Autodesk Fusion 360 part; units mm, degrees
(part 3 of 4)
sketch "v3" plane through (0, 0, 0) normal (0, 1, 0) x (1, 0, 0)
  line L0 (97.775, -35.41) -> (97.775, -48.41)
  arc A0 (111.775, -54.46) -> (111.275, -53.96) centre (111.275, -54.46) ccw
  arc A1 (68.5566, -88.749) -> (70.5283, -89.9625) centre (70.9931, -86.9987) ccw
  arc A2 (98.275, -34.91) -> (97.775, -35.41) centre (98.275, -35.41) ccw
  arc A3 (92.725, -52.555) -> (92.225, -52.055) centre (92.225, -52.555) ccw
  arc A4 (79.225, -52.055) -> (78.725, -52.555) centre (79.225, -52.555) ccw
  arc A5 (92.225, -47.005) -> (92.725, -46.505) centre (92.225, -46.505) ccw
  arc A6 (73.175, -56.53) -> (73.675, -56.03) centre (73.175, -56.03) ccw
  line L1 (92.225, -52.555) -> (92.225, -46.505) construction
  line L2 (79.225, -47.005) -> (92.225, -47.005)
  arc A7 (2.525, -73.175) -> (3.025, -73.675) centre (3.025, -73.175) ccw
  line L3 (113.775, -14.86) -> (113.775, -16.36)
  arc A8 (54.125, -24.145) -> (54.625, -23.645) centre (54.125, -23.645) ccw
  line L4 (22.075, -33.67) -> (35.075, -33.67)
  arc A9 (111.775, -16.36) -> (111.275, -15.86) centre (111.275, -16.36) ccw
  arc A10 (73.175, -18.43) -> (73.675, -17.93) centre (73.175, -17.93) ccw
  arc A11 (40.625, -42.695) -> (41.125, -43.195) centre (41.125, -42.695) ccw
  line L5 (35.575, -20.17) -> (35.575, -33.17)
  arc A12 (21.575, -33.17) -> (22.075, -33.67) centre (22.075, -33.17) ccw
  arc A13 (120.896, -78.4821) -> (120.213, -78.6651) centre (120.646, -78.9151) ccw
  line L6 (40.625, -10.645) -> (40.625, -23.645)
  line L7 (59.675, -23.98) -> (59.675, -36.98)
  line L8 (79.225, -66.055) -> (92.225, -66.055)
  arc A14 (113.775, -14.86) -> (112.775, -13.86) centre (112.775, -14.86) ccw
  arc A15 (40.625, -61.745) -> (41.125, -62.245) centre (41.125, -61.745) ccw
  line L9 (68.5566, -88.749) -> (60.0623, -76.9247)
  line L10 (22.075, -35.075) -> (22.075, -41.125) construction
  line L11 (22.075, -41.125) -> (16.025, -41.125) construction
  arc A16 (109.3213, -79.6939) -> (108.9677, -79.0815) centre (108.8383, -79.5645) ccw
  line L12 (22.075, -57.77) -> (35.075, -57.77)
  arc A17 (113.775, -65.0177) -> (115.275, -67.6158) centre (116.775, -65.0177) ccw
  arc A18 (41.125, -29.195) -> (40.625, -29.695) centre (41.125, -29.695) ccw
  line L13 (41.125, -43.195) -> (54.125, -43.195)
  arc A19 (94.725, -13.36) -> (95.225, -13.86) centre (95.225, -13.36) ccw
  arc A20 (35.575, -39.22) -> (35.075, -38.72) centre (35.075, -39.22) ccw
  arc A21 (40.625, -23.645) -> (41.125, -24.145) centre (41.125, -23.645) ccw
  arc A22 (92.4336, -88.6274) -> (92.7872, -89.2398) centre (92.9166, -88.7568) ccw
  line L14 (136.7533, -80.0163) -> (115.275, -67.6158)
  arc A23 (54.125, -62.245) -> (54.625, -61.745) centre (54.125, -61.745) ccw
  line L15 (21.575, -20.17) -> (21.575, -33.17)
  line L16 (22.075, -19.67) -> (35.075, -19.67)
  arc A24 (60.175, -23.48) -> (59.675, -23.98) centre (60.175, -23.98) ccw
  line L17 (94.725, -12.455) -> (94.725, -13.36)
  arc A25 (92.225, -66.055) -> (92.725, -65.555) centre (92.225, -65.555) ccw
  line L18 (73.675, -4.93) -> (73.675, -17.93)
  arc A26 (60.175, -4.43) -> (59.675, -4.93) centre (60.175, -4.93) ccw
  arc A27 (85.5575, -87.9625) -> (86.0575, -87.4625) centre (85.5575, -87.4625) ccw
  arc A28 (3.025, -40.625) -> (2.525, -41.125) centre (3.025, -41.125) ccw
  line L19 (35.575, -58.27) -> (35.575, -71.27)
  line L20 (75.175, -2.43) -> (73.175, -2.43)
  arc A29 (3.025, -21.575) -> (2.525, -22.075) centre (3.025, -22.075) ccw
  line L21 (107.725, -13.86) -> (112.775, -13.86)
  line L22 (57.675, -7.645) -> (57.675, -2.93)
  arc A30 (54.625, -48.745) -> (54.125, -48.245) centre (54.125, -48.745) ccw
  arc A31 (94.725, -12.455) -> (94.225, -11.955) centre (94.225, -12.455) ccw
  arc A32 (57.175, -8.145) -> (57.675, -7.645) centre (57.175, -7.645) ccw
  arc A33 (2.525, -54.125) -> (3.025, -54.625) centre (3.025, -54.125) ccw
  arc A34 (60.175, -42.53) -> (59.675, -43.03) centre (60.175, -43.03) ccw
  line L23 (41.125, -24.145) -> (54.125, -24.145)
  circle A35 centre (66.675, -65.625) radius 1
  line L24 (120.213, -78.6651) -> (113.713, -89.9234)
  line L25 (3.025, -54.625) -> (16.025, -54.625)
  arc A36 (54.625, -10.645) -> (54.125, -10.145) centre (54.125, -10.645) ccw
  line L26 (125.1543, -97.1064) -> (113.896, -90.6064)
  line L27 (72.5575, -73.9625) -> (85.5575, -73.9625)
  line L28 (3.025, -35.575) -> (16.025, -35.575)
  arc A37 (73.675, -4.93) -> (73.175, -4.43) centre (73.175, -4.93) ccw
  arc A38 (54.625, -29.695) -> (54.125, -29.195) centre (54.125, -29.695) ccw
  line L29 (86.0575, -74.4625) -> (86.0575, -87.4625)
  arc A39 (35.075, -33.67) -> (35.575, -33.17) centre (35.075, -33.17) ccw
  line L30 (22.075, -38.72) -> (35.075, -38.72)
  arc A40 (132.3373, -85.6651) -> (132.1543, -84.9821) centre (131.9043, -85.4151) ccw
  line L31 (0.525, -22.075) -> (0.525, -35.075)
  line L32 (41.125, -29.195) -> (54.125, -29.195)
  arc A41 (79.225, -13.955) -> (78.725, -14.455) centre (79.225, -14.455) ccw
  line L33 (54.625, -29.695) -> (54.625, -42.695)
  line L34 (70.5283, -89.9625) -> (109.8625, -96.1307)
  line L35 (59.675, -43.03) -> (59.675, -56.03)
  line L36 (25.625, -17.67) -> (38.125, -17.67)
  line L37 (92.7872, -89.2398) -> (105.3442, -92.6045)
  line L38 (98.275, -67.96) -> (111.275, -67.96)
  circle A42 centre (95.25, -49.53) radius 1
  line L39 (113.775, -16.36) -> (113.775, -29.36)
  line L40 (97.775, -54.46) -> (97.775, -67.46)
  line L41 (95.7983, -76.0704) -> (92.4336, -88.6274)
  line L42 (92.725, -14.455) -> (92.725, -27.455)
  line L43 (16.025, -35.075) -> (22.075, -35.075) construction
  line L44 (73.675, -23.98) -> (73.675, -36.98)
  line L45 (132.1543, -84.9821) -> (120.896, -78.4821)
  line L46 (22.075, -71.77) -> (35.075, -71.77)
  line L47 (0.525, -41.125) -> (0.525, -54.125)
  line L48 (16.525, -41.125) -> (16.525, -54.125)
  line L49 (98.275, -33.505) -> (92.225, -33.505) construction
  line L50 (2.525, -41.125) -> (2.525, -54.125)
  line L51 (97.775, -16.36) -> (97.775, -29.36)
  line L52 (40.625, -29.695) -> (40.625, -42.695)
  line L53 (111.775, -16.36) -> (111.775, -29.36)
  line L54 (98.275, -52.555) -> (92.225, -52.555) construction
  line L55 (22.075, -52.72) -> (35.075, -52.72)
  line L56 (78.725, -14.455) -> (78.725, -27.455)
  line L57 (92.225, -27.455) -> (98.275, -27.455) construction
  line L58 (96.4107, -75.7169) -> (108.9677, -79.0815)
  line L59 (132.1543, -84.9821) -> (120.896, -78.4821)
  line L60 (20.075, -17.67) -> (25.625, -17.67)
  arc A43 (137.1194, -81.3823) -> (136.7533, -80.0163) centre (136.2533, -80.8823) ccw
  line L61 (88.675, -11.955) -> (94.225, -11.955)
  line L62 (22.075, -71.77) -> (35.075, -71.77)
  arc A44 (111.275, -67.96) -> (111.775, -67.46) centre (111.275, -67.46) ccw
  arc A45 (97.775, -67.46) -> (98.275, -67.96) centre (98.275, -67.46) ccw
  line L63 (54.625, -10.645) -> (54.625, -23.645)
  line L64 (16.025, -75.675) -> (57.6258, -75.675)
  line L65 (39.125, -8.145) -> (44.675, -8.145)
  arc A46 (35.575, -58.27) -> (35.075, -57.77) centre (35.075, -58.27) ccw
  arc A47 (41.125, -10.145) -> (40.625, -10.645) centre (41.125, -10.645) ccw
  line L66 (19.575, -19.075) -> (19.575, -18.17)
  arc A48 (19.075, -19.575) -> (19.575, -19.075) centre (19.075, -19.075) ccw
  line L67 (41.125, -48.245) -> (54.125, -48.245)
  line L68 (58.175, -2.43) -> (60.175, -2.43)
  arc A49 (16.525, -22.075) -> (16.025, -21.575) centre (16.025, -22.075) ccw
  line L69 (40.625, -48.745) -> (40.625, -61.745)
  arc A50 (41.125, -48.245) -> (40.625, -48.745) centre (41.125, -48.745) ccw
  line L70 (137.1194, -81.3823) -> (127.5694, -97.9234)
  circle A51 centre (19.05, -38.1) radius 1
  line L71 (22.075, -54.125) -> (22.075, -60.175) construction
  arc A52 (125.1543, -97.1064) -> (125.8373, -96.9234) centre (125.4043, -96.6734) ccw
  arc A53 (123.1533, -103.5722) -> (124.5194, -103.2062) centre (123.6533, -102.7062) ccw
  line L72 (132.3373, -85.6651) -> (125.8373, -96.9234)
  arc A54 (16.525, -41.125) -> (16.025, -40.625) centre (16.025, -41.125) ccw
  line L73 (0.525, -60.175) -> (0.525, -74.675)
  arc A55 (21.575, -52.22) -> (22.075, -52.72) centre (22.075, -52.22) ccw
  line L74 (2.525, -60.175) -> (2.525, -73.175)
  arc A56 (16.525, -60.175) -> (16.025, -59.675) centre (16.025, -60.175) ccw
  arc A57 (75.675, -11.455) -> (76.175, -11.955) centre (76.175, -11.455) ccw
  line L75 (16.025, -41.125) -> (16.025, -35.075) construction
  line L76 (0.525, -22.075) -> (0.525, -20.575)
  line L77 (2.525, -22.075) -> (2.525, -35.075)
  line L78 (54.625, -48.745) -> (54.625, -61.745)
  line L79 (6.575, -19.575) -> (19.075, -19.575)
  line L80 (16.525, -60.175) -> (16.525, -73.175)
  arc A58 (35.075, -71.77) -> (35.575, -71.27) centre (35.075, -71.27) ccw
  line L81 (22.075, -60.175) -> (16.025, -60.175) construction
  line L82 (3.025, -73.675) -> (16.025, -73.675)
  line L83 (0.525, -60.175) -> (0.525, -54.125)
  line L84 (16.025, -60.175) -> (16.025, -54.125) construction
  line L85 (3.025, -21.575) -> (16.025, -21.575)
  arc A59 (16.025, -73.675) -> (16.525, -73.175) centre (16.025, -73.175) ccw
  line L86 (1.525, -19.575) -> (3.025, -19.575)
  arc A60 (21.575, -71.27) -> (22.075, -71.77) centre (22.075, -71.27) ccw
  line L87 (6.575, -19.575) -> (3.025, -19.575)
  line L88 (2.525, -60.175) -> (2.525, -73.175)
  arc A61 (3.025, -59.675) -> (2.525, -60.175) centre (3.025, -60.175) ccw
  arc A62 (0.525, -74.675) -> (1.525, -75.675) centre (1.525, -74.675) ccw
  line L89 (1.525, -75.675) -> (16.025, -75.675)
  arc A63 (1.525, -19.575) -> (0.525, -20.575) centre (1.525, -20.575) ccw
  arc A64 (20.075, -17.67) -> (19.575, -18.17) centre (20.075, -18.17) ccw
  arc A65 (78.725, -65.555) -> (79.225, -66.055) centre (79.225, -65.555) ccw
  arc A66 (16.025, -35.575) -> (16.525, -35.075) centre (16.025, -35.075) ccw
  line L90 (75.675, -11.455) -> (75.675, -2.93)
  arc A67 (39.125, -8.145) -> (38.625, -8.645) centre (39.125, -8.645) ccw
  line L91 (0.525, -41.125) -> (0.525, -35.075)
  line L92 (59.675, -4.93) -> (59.675, -17.93)
  arc A68 (113.713, -89.9234) -> (113.896, -90.6064) centre (114.146, -90.1734) ccw
  arc A69 (72.0575, -87.4625) -> (72.5575, -87.9625) centre (72.5575, -87.4625) ccw
  arc A70 (22.075, -38.72) -> (21.575, -39.22) centre (22.075, -39.22) ccw
  arc A71 (59.675, -36.98) -> (60.175, -37.48) centre (60.175, -36.98) ccw
  arc A72 (22.075, -19.67) -> (21.575, -20.17) centre (22.075, -20.17) ccw
  arc A73 (59.675, -17.93) -> (60.175, -18.43) centre (60.175, -17.93) ccw
  arc A74 (16.025, -54.625) -> (16.525, -54.125) centre (16.025, -54.125) ccw
  arc A75 (38.125, -17.67) -> (38.625, -17.17) centre (38.125, -17.17) ccw
  arc A76 (35.075, -52.72) -> (35.575, -52.22) centre (35.075, -52.22) ccw
  line L93 (38.625, -17.17) -> (38.625, -8.645)
  arc A77 (86.0575, -74.4625) -> (85.5575, -73.9625) centre (85.5575, -74.4625) ccw
  line L94 (41.125, -62.245) -> (54.125, -62.245)
  line L95 (72.0575, -74.4625) -> (72.0575, -87.4625)
  arc A78 (60.0623, -76.9247) -> (57.6258, -75.675) centre (57.6258, -78.675) ccw
  circle A79 centre (19.05, -57.15) radius 1
  line L96 (76.175, -11.955) -> (88.675, -11.955)
  line L97 (41.125, -62.245) -> (54.125, -62.245)
  line L98 (123.1533, -103.5722) -> (110.8977, -96.4964)
  line L99 (44.675, -8.145) -> (57.175, -8.145)
  line L100 (72.0575, -74.4625) -> (72.0575, -87.4625)
  arc A80 (22.075, -57.77) -> (21.575, -58.27) centre (22.075, -58.27) ccw
  line L101 (3.025, -40.625) -> (16.025, -40.625)
  arc A81 (105.3442, -92.6045) -> (105.9566, -92.2509) centre (105.4736, -92.1215) ccw
  arc A82 (35.575, -20.17) -> (35.075, -19.67) centre (35.075, -20.17) ccw
  arc A83 (98.275, -15.86) -> (97.775, -16.36) centre (98.275, -16.36) ccw
  line L102 (79.225, -13.955) -> (92.225, -13.955)
  line L103 (109.3213, -79.6939) -> (105.9566, -92.2509)
  line L104 (98.275, -15.86) -> (111.275, -15.86)
  arc A84 (59.675, -56.03) -> (60.175, -56.53) centre (60.175, -56.03) ccw
  arc A85 (96.4107, -75.7169) -> (95.7983, -76.0704) centre (96.2813, -76.1998) ccw
  line L105 (41.125, -10.145) -> (54.125, -10.145)
  line L106 (16.025, -54.125) -> (22.075, -54.125) construction
  line L107 (21.575, -58.27) -> (21.575, -71.27)
  arc A86 (110.8977, -96.4964) -> (109.8625, -96.1307) centre (109.3977, -99.0945) ccw
  line L108 (95.225, -13.86) -> (107.725, -13.86)
  line L109 (16.525, -22.075) -> (16.525, -35.075)
  arc A87 (54.125, -43.195) -> (54.625, -42.695) centre (54.125, -42.695) ccw
  arc A88 (72.5575, -73.9625) -> (72.0575, -74.4625) centre (72.5575, -74.4625) ccw
  line L110 (3.025, -59.675) -> (16.025, -59.675)
  arc A89 (2.525, -35.075) -> (3.025, -35.575) centre (3.025, -35.075) ccw
  line L111 (72.5575, -87.9625) -> (85.5575, -87.9625)
  line L112 (124.5194, -103.2062) -> (127.5694, -97.9234)
  arc A90 (92.725, -14.455) -> (92.225, -13.955) centre (92.225, -14.455) ccw
  arc A91 (75.675, -2.93) -> (75.175, -2.43) centre (75.175, -2.93) ccw
  line L113 (66.675, -47.625) -> (66.675, -65.625) construction
  arc A92 (58.175, -2.43) -> (57.675, -2.93) centre (58.175, -2.93) ccw
  arc A93 (73.675, -23.98) -> (73.175, -23.48) centre (73.175, -23.98) ccw
  arc A94 (111.275, -48.91) -> (111.775, -48.41) centre (111.275, -48.41) ccw
  arc A95 (97.775, -29.36) -> (98.275, -29.86) centre (98.275, -29.36) ccw
  line L114 (98.275, -27.455) -> (98.275, -33.505) construction
  line L115 (111.775, -35.41) -> (111.775, -48.41)
  arc A96 (111.275, -29.86) -> (111.775, -29.36) centre (111.275, -29.36) ccw
  line L116 (98.275, -29.86) -> (111.275, -29.86)
  line L117 (98.275, -46.505) -> (98.275, -52.555) construction
  line L118 (98.275, -53.96) -> (111.275, -53.96)
  line L119 (98.275, -48.91) -> (111.275, -48.91)
  line L120 (98.275, -34.91) -> (111.275, -34.91)
  line L121 (113.775, -54.46) -> (113.775, -48.41)
  arc A97 (98.275, -53.96) -> (97.775, -54.46) centre (98.275, -54.46) ccw
  line L122 (113.775, -35.41) -> (113.775, -29.36)
  arc A98 (111.775, -35.41) -> (111.275, -34.91) centre (111.275, -35.41) ccw
  line L123 (113.775, -35.41) -> (113.775, -48.41)
  arc A99 (97.775, -48.41) -> (98.275, -48.91) centre (98.275, -48.41) ccw
  line L124 (79.225, -27.955) -> (92.225, -27.955)
  arc A100 (78.725, -27.455) -> (79.225, -27.955) centre (79.225, -27.455) ccw
  line L125 (79.225, -33.005) -> (92.225, -33.005)
  line L126 (60.175, -2.43) -> (73.175, -2.43)
  arc A101 (79.225, -33.005) -> (78.725, -33.505) centre (79.225, -33.505) ccw
  line L127 (113.775, -54.46) -> (113.775, -65.0177)
  line L128 (92.725, -52.555) -> (92.725, -65.555)
  line L129 (2.525, -41.125) -> (2.525, -54.125)
  line L130 (78.725, -52.555) -> (78.725, -65.555)
  line L131 (92.225, -33.505) -> (92.225, -27.455) construction
  line L132 (92.225, -46.505) -> (98.275, -46.505) construction
  circle A102 centre (95.25, -30.48) radius 1
  line L133 (111.775, -54.46) -> (111.775, -67.46)
  arc A103 (92.225, -27.955) -> (92.725, -27.455) centre (92.225, -27.455) ccw
  line L134 (73.675, -43.03) -> (73.675, -56.03)
  line L135 (35.575, -39.22) -> (35.575, -52.22)
  line L136 (21.575, -39.22) -> (21.575, -52.22)
  line L137 (60.175, -18.43) -> (73.175, -18.43)
  arc A104 (92.725, -33.505) -> (92.225, -33.005) centre (92.225, -33.505) ccw
  line L138 (60.175, -23.48) -> (73.175, -23.48)
  line L139 (79.225, -52.055) -> (92.225, -52.055)
  line L140 (78.725, -33.505) -> (78.725, -46.505)
  arc A105 (73.175, -37.48) -> (73.675, -36.98) centre (73.175, -36.98) ccw
  arc A106 (78.725, -46.505) -> (79.225, -47.005) centre (79.225, -46.505) ccw
  line L141 (60.175, -37.48) -> (73.175, -37.48)
  line L142 (60.175, -42.53) -> (73.175, -42.53)
  arc A107 (73.675, -43.03) -> (73.175, -42.53) centre (73.175, -43.03) ccw
  line L143 (60.175, -56.53) -> (73.175, -56.53)
  line L144 (60.175, -4.43) -> (73.175, -4.43)
  line L145 (92.725, -33.505) -> (92.725, -46.505)
  line L146 (150, 0) -> (150, -125) construction
  line L147 (179.787, -78.6651) -> (186.287, -89.9234)
  line L148 (167.8457, -84.9821) -> (179.104, -78.4821)
  line L149 (190.6787, -79.6939) -> (194.0434, -92.2509)
  line L150 (162.8806, -81.3823) -> (172.4306, -97.9234)
  line L151 (167.8457, -84.9821) -> (179.104, -78.4821)
  line L152 (239.825, -4.43) -> (226.825, -4.43)
  line L153 (239.825, -2.43) -> (226.825, -2.43)
  arc A108 (204.2017, -76.0704) -> (203.5893, -75.7169) centre (203.7187, -76.1998) ccw
  arc A109 (207.2128, -89.2398) -> (207.5664, -88.6274) centre (207.0834, -88.7568) ccw
  line L154 (239.825, -42.53) -> (226.825, -42.53)
  arc A110 (229.4717, -89.9625) -> (231.4434, -88.749) centre (229.0069, -86.9987) ccw
  arc A111 (207.275, -65.555) -> (207.775, -66.055) centre (207.775, -65.555) ccw
  arc A112 (213.9425, -87.4625) -> (214.4425, -87.9625) centre (214.4425, -87.4625) ccw
  circle A113 centre (204.75, -49.53) radius 1
  arc A114 (202.225, -16.36) -> (201.725, -15.86) centre (201.725, -16.36) ccw
  line L155 (201.725, -27.455) -> (201.725, -33.505) construction
  line L156 (205.275, -12.455) -> (205.275, -13.36)
  line L157 (226.325, -43.03) -> (226.325, -56.03)
  line L158 (224.325, -11.455) -> (224.325, -2.93)
  arc A115 (188.725, -15.86) -> (188.225, -16.36) centre (188.725, -16.36) ccw
  arc A116 (205.775, -11.955) -> (205.275, -12.455) centre (205.775, -12.455) ccw
  arc A117 (207.275, -27.455) -> (207.775, -27.955) centre (207.775, -27.455) ccw
  arc A118 (204.775, -13.86) -> (205.275, -13.36) centre (204.775, -13.36) ccw
  line L159 (207.775, -27.455) -> (201.725, -27.455) construction
  line L160 (220.775, -47.005) -> (207.775, -47.005)
  line L161 (188.225, -35.41) -> (188.225, -48.41)
  line L162 (192.275, -13.86) -> (187.225, -13.86)
  line L163 (298.475, -19.575) -> (296.975, -19.575)
  arc A119 (259.375, -48.745) -> (258.875, -48.245) centre (258.875, -48.745) ccw
  line L164 (201.725, -15.86) -> (188.725, -15.86)
  line L165 (283.475, -60.175) -> (283.475, -73.175)
  arc A120 (201.725, -48.91) -> (202.225, -48.41) centre (201.725, -48.41) ccw
  line L166 (298.475, -75.675) -> (283.975, -75.675)
  arc A121 (188.725, -53.96) -> (188.225, -54.46) centre (188.725, -54.46) ccw
  line L167 (186.225, -14.86) -> (186.225, -16.36)
  arc A122 (187.225, -13.86) -> (186.225, -14.86) centre (187.225, -14.86) ccw
  line L168 (299.475, -60.175) -> (299.475, -74.675)
  line L169 (201.725, -53.96) -> (188.725, -53.96)
  line L170 (224.825, -2.43) -> (226.825, -2.43)
  line L171 (226.325, -4.93) -> (226.325, -17.93)
  arc A123 (201.725, -29.86) -> (202.225, -29.36) centre (201.725, -29.36) ccw
  arc A124 (226.825, -23.48) -> (226.325, -23.98) centre (226.825, -23.98) ccw
  arc A125 (224.825, -2.43) -> (224.325, -2.93) centre (224.825, -2.93) ccw
  line L172 (223.825, -11.955) -> (211.325, -11.955)
  arc A126 (277.925, -52.72) -> (278.425, -52.22) centre (277.925, -52.22) ccw
  arc A127 (207.275, -46.505) -> (207.775, -47.005) centre (207.775, -46.505) ccw
  line L173 (201.725, -34.91) -> (188.725, -34.91)
  arc A128 (226.825, -4.43) -> (226.325, -4.93) centre (226.825, -4.93) ccw
  arc A129 (223.825, -11.955) -> (224.325, -11.455) centre (223.825, -11.455) ccw
  circle A130 centre (280.95, -57.15) radius 1
  line L174 (201.725, -46.505) -> (201.725, -52.555) construction
  line L175 (283.975, -54.125) -> (277.925, -54.125) construction
  line L176 (220.775, -52.055) -> (207.775, -52.055)
  line L177 (220.775, -13.955) -> (207.775, -13.955)
  arc A131 (207.775, -13.955) -> (207.275, -14.455) centre (207.775, -14.455) ccw
  line L178 (296.975, -59.675) -> (283.975, -59.675)
  line L179 (296.975, -54.625) -> (283.975, -54.625)
  arc A132 (221.275, -14.455) -> (220.775, -13.955) centre (220.775, -14.455) ccw
  arc A133 (226.325, -17.93) -> (226.825, -18.43) centre (226.825, -17.93) ccw
  line L180 (207.275, -33.505) -> (207.275, -46.505)
  arc A134 (296.975, -54.625) -> (297.475, -54.125) centre (296.975, -54.125) ccw
  arc A135 (226.825, -42.53) -> (226.325, -43.03) centre (226.825, -43.03) ccw
  arc A136 (283.475, -54.125) -> (283.975, -54.625) centre (283.975, -54.125) ccw
  arc A137 (220.775, -27.955) -> (221.275, -27.455) centre (220.775, -27.455) ccw
  arc A138 (278.425, -58.27) -> (277.925, -57.77) centre (277.925, -58.27) ccw
  arc A139 (283.475, -73.175) -> (283.975, -73.675) centre (283.975, -73.175) ccw
  arc A140 (239.825, -56.53) -> (240.325, -56.03) centre (239.825, -56.03) ccw
  arc A141 (280.425, -18.17) -> (279.925, -17.67) centre (279.925, -18.17) ccw
  line L181 (201.725, -33.505) -> (207.775, -33.505) construction
  line L182 (186.225, -35.41) -> (186.225, -29.36)
  line L183 (299.475, -22.075) -> (299.475, -35.075)
  arc A142 (299.475, -20.575) -> (298.475, -19.575) centre (298.475, -20.575) ccw
  circle A143 centre (280.95, -38.1) radius 1
  line L184 (277.925, -60.175) -> (283.975, -60.175) construction
  circle A144 centre (204.75, -30.48) radius 1
  line L185 (297.475, -22.075) -> (297.475, -35.075)
  line L186 (201.725, -52.555) -> (207.775, -52.555) construction
  arc A145 (283.475, -35.075) -> (283.975, -35.575) centre (283.975, -35.075) ccw
  line L187 (280.425, -19.075) -> (280.425, -18.17)
  arc A146 (240.325, -43.03) -> (239.825, -42.53) centre (239.825, -43.03) ccw
  line L188 (293.425, -19.575) -> (280.925, -19.575)
  arc A147 (202.225, -35.41) -> (201.725, -34.91) centre (201.725, -35.41) ccw
  line L189 (296.975, -73.675) -> (283.975, -73.675)
  line L190 (264.425, -58.27) -> (264.425, -71.27)
  line L191 (231.4434, -88.749) -> (239.9377, -76.9247)
  line L192 (258.875, -62.245) -> (245.875, -62.245)
  line L193 (283.975, -60.175) -> (283.975, -54.125) construction
  line L194 (299.475, -41.125) -> (299.475, -35.075)
  arc A148 (280.425, -19.075) -> (280.925, -19.575) centre (280.925, -19.075) ccw
  line L195 (211.325, -11.955) -> (205.775, -11.955)
  line L196 (296.975, -21.575) -> (283.975, -21.575)
  line L197 (283.975, -41.125) -> (283.975, -35.075) construction
  line L198 (283.475, -22.075) -> (283.475, -35.075)
  arc A149 (245.875, -48.245) -> (245.375, -48.745) centre (245.875, -48.745) ccw
  line L199 (186.225, -54.46) -> (186.225, -48.41)
  arc A150 (296.975, -73.675) -> (297.475, -73.175) centre (296.975, -73.175) ccw
  line L200 (233.325, -47.625) -> (233.325, -65.625) construction
  line L201 (278.425, -58.27) -> (278.425, -71.27)
  arc A151 (298.475, -75.675) -> (299.475, -74.675) centre (298.475, -74.675) ccw
  line L202 (207.775, -46.505) -> (201.725, -46.505) construction
  line L203 (204.775, -13.86) -> (192.275, -13.86)
  line L204 (258.875, -62.245) -> (245.875, -62.245)
  line L205 (186.225, -35.41) -> (186.225, -48.41)
  line L206 (201.725, -48.91) -> (188.725, -48.91)
  line L207 (293.425, -19.575) -> (296.975, -19.575)
  line L208 (277.925, -54.125) -> (277.925, -60.175) construction
  line L209 (258.875, -10.145) -> (245.875, -10.145)
  line L210 (277.925, -52.72) -> (264.925, -52.72)
  line L211 (259.375, -10.645) -> (259.375, -23.645)
  line L212 (274.375, -17.67) -> (261.875, -17.67)
  line L213 (229.4717, -89.9625) -> (190.1375, -96.1307)
  arc A152 (258.875, -24.145) -> (259.375, -23.645) centre (258.875, -23.645) ccw
  line L214 (283.975, -35.075) -> (277.925, -35.075) construction
  line L215 (258.875, -29.195) -> (245.875, -29.195)
  line L216 (279.925, -17.67) -> (274.375, -17.67)
  arc A153 (245.875, -10.145) -> (245.375, -10.645) centre (245.875, -10.645) ccw
  line L217 (259.375, -48.745) -> (259.375, -61.745)
  arc A154 (239.825, -37.48) -> (240.325, -36.98) centre (239.825, -36.98) ccw
  line L218 (277.925, -57.77) -> (264.925, -57.77)
  line L219 (258.875, -24.145) -> (245.875, -24.145)
  line L220 (207.2128, -89.2398) -> (194.6558, -92.6045)
  line L221 (241.825, -2.43) -> (239.825, -2.43)
  line L222 (255.325, -8.145) -> (242.825, -8.145)
  arc A155 (240.325, -4.93) -> (239.825, -4.43) centre (239.825, -4.93) ccw
  line L223 (245.375, -10.645) -> (245.375, -23.645)
  arc A156 (258.875, -62.245) -> (259.375, -61.745) centre (258.875, -61.745) ccw
  line L224 (202.225, -16.36) -> (202.225, -29.36)
  line L225 (277.925, -41.125) -> (283.975, -41.125) construction
  arc A157 (245.375, -23.645) -> (245.875, -24.145) centre (245.875, -23.645) ccw
  arc A158 (245.875, -29.195) -> (245.375, -29.695) centre (245.875, -29.695) ccw
  line L226 (283.975, -75.675) -> (242.3742, -75.675)
  arc A159 (259.375, -29.695) -> (258.875, -29.195) centre (258.875, -29.695) ccw
  arc A160 (245.375, -42.695) -> (245.875, -43.195) centre (245.875, -42.695) ccw
  arc A161 (283.975, -21.575) -> (283.475, -22.075) centre (283.975, -22.075) ccw
  arc A162 (240.325, -23.98) -> (239.825, -23.48) centre (239.825, -23.98) ccw
  line L227 (240.325, -43.03) -> (240.325, -56.03)
  arc A163 (242.325, -2.93) -> (241.825, -2.43) centre (241.825, -2.93) ccw
  line L228 (277.925, -71.77) -> (264.925, -71.77)
  arc A164 (242.3742, -75.675) -> (239.9377, -76.9247) centre (242.3742, -78.675) ccw
  line L229 (277.925, -19.67) -> (264.925, -19.67)
  arc A165 (239.825, -18.43) -> (240.325, -17.93) centre (239.825, -17.93) ccw
  line L230 (299.475, -22.075) -> (299.475, -20.575)
  arc A166 (277.925, -33.67) -> (278.425, -33.17) centre (277.925, -33.17) ccw
  line L231 (240.325, -23.98) -> (240.325, -36.98)
  line L232 (277.925, -35.075) -> (277.925, -41.125) construction
  line L233 (242.325, -7.645) -> (242.325, -2.93)
  arc A167 (264.425, -33.17) -> (264.925, -33.67) centre (264.925, -33.17) ccw
  arc A168 (264.925, -38.72) -> (264.425, -39.22) centre (264.925, -39.22) ccw
  line L234 (261.375, -17.17) -> (261.375, -8.645)
  arc A169 (264.925, -19.67) -> (264.425, -20.17) centre (264.925, -20.17) ccw
  arc A170 (297.475, -60.175) -> (296.975, -59.675) centre (296.975, -60.175) ccw
  line L235 (240.325, -4.93) -> (240.325, -17.93)
  arc A171 (259.375, -10.645) -> (258.875, -10.145) centre (258.875, -10.645) ccw
  arc A172 (245.375, -61.745) -> (245.875, -62.245) centre (245.875, -61.745) ccw
  line L236 (264.425, -20.17) -> (264.425, -33.17)
  arc A173 (202.225, -54.46) -> (201.725, -53.96) centre (201.725, -54.46) ccw
  arc A174 (258.875, -43.195) -> (259.375, -42.695) centre (258.875, -42.695) ccw
  arc A175 (264.425, -71.27) -> (264.925, -71.77) centre (264.925, -71.27) ccw
  arc A176 (297.475, -41.125) -> (296.975, -40.625) centre (296.975, -41.125) ccw
  arc A177 (261.375, -17.17) -> (261.875, -17.67) centre (261.875, -17.17) ccw
  line L237 (258.875, -48.245) -> (245.875, -48.245)
  line L238 (277.925, -38.72) -> (264.925, -38.72)
  line L239 (245.375, -48.745) -> (245.375, -61.745)
  line L240 (278.425, -20.17) -> (278.425, -33.17)
  line L241 (226.325, -23.98) -> (226.325, -36.98)
  line L242 (260.875, -8.145) -> (255.325, -8.145)
  circle A178 centre (233.325, -65.625) radius 1
  arc A179 (296.975, -35.575) -> (297.475, -35.075) centre (296.975, -35.075) ccw
  line L243 (202.225, -35.41) -> (202.225, -48.41)
  arc A180 (297.475, -22.075) -> (296.975, -21.575) centre (296.975, -22.075) ccw
  line L244 (297.475, -60.175) -> (297.475, -73.175)
  arc A181 (278.425, -20.17) -> (277.925, -19.67) centre (277.925, -20.17) ccw
  arc A182 (242.325, -7.645) -> (242.825, -8.145) centre (242.825, -7.645) ccw
  arc A183 (188.725, -34.91) -> (188.225, -35.41) centre (188.725, -35.41) ccw
  line L245 (297.475, -60.175) -> (297.475, -73.175)
  arc A184 (261.375, -8.645) -> (260.875, -8.145) centre (260.875, -8.645) ccw
  arc A185 (278.425, -39.22) -> (277.925, -38.72) centre (277.925, -39.22) ccw
  line L246 (296.975, -35.575) -> (283.975, -35.575)
  arc A186 (188.225, -48.41) -> (188.725, -48.91) centre (188.725, -48.41) ccw
  line L247 (299.475, -60.175) -> (299.475, -54.125)
  arc A187 (264.925, -57.77) -> (264.425, -58.27) centre (264.925, -58.27) ccw
  arc A188 (283.975, -40.625) -> (283.475, -41.125) centre (283.975, -41.125) ccw
  arc A189 (188.225, -29.36) -> (188.725, -29.86) centre (188.725, -29.36) ccw
  line L248 (221.275, -14.455) -> (221.275, -27.455)
  arc A190 (264.425, -52.22) -> (264.925, -52.72) centre (264.925, -52.22) ccw
  line L249 (188.225, -16.36) -> (188.225, -29.36)
  line L250 (296.975, -40.625) -> (283.975, -40.625)
  arc A191 (283.975, -59.675) -> (283.475, -60.175) centre (283.975, -60.175) ccw
  arc A192 (277.925, -71.77) -> (278.425, -71.27) centre (277.925, -71.27) ccw
  line L251 (201.725, -29.86) -> (188.725, -29.86)
  line L252 (277.925, -33.67) -> (264.925, -33.67)
  line L253 (258.875, -43.195) -> (245.875, -43.195)
  arc A193 (221.275, -52.555) -> (220.775, -52.055) centre (220.775, -52.555) ccw
  line L254 (220.775, -33.005) -> (207.775, -33.005)
  line L255 (220.775, -27.955) -> (207.775, -27.955)
  arc A194 (221.275, -33.505) -> (220.775, -33.005) centre (220.775, -33.505) ccw
  line L256 (207.775, -52.555) -> (207.775, -46.505) construction
  arc A195 (226.325, -36.98) -> (226.825, -37.48) centre (226.825, -36.98) ccw
  arc A196 (220.775, -47.005) -> (221.275, -46.505) centre (220.775, -46.505) ccw
  arc A197 (207.775, -52.055) -> (207.275, -52.555) centre (207.775, -52.555) ccw
  line L257 (207.775, -33.505) -> (207.775, -27.455) construction
  arc A198 (207.775, -33.005) -> (207.275, -33.505) centre (207.775, -33.505) ccw
  arc A199 (226.325, -56.03) -> (226.825, -56.53) centre (226.825, -56.03) ccw
  line L258 (221.275, -33.505) -> (221.275, -46.505)
  line L259 (227.9425, -74.4625) -> (227.9425, -87.4625)
  arc A200 (227.4425, -87.9625) -> (227.9425, -87.4625) centre (227.4425, -87.4625) ccw
  arc A201 (201.725, -67.96) -> (202.225, -67.46) centre (201.725, -67.46) ccw
  line L260 (227.4425, -73.9625) -> (214.4425, -73.9625)
  line L261 (239.825, -56.53) -> (226.825, -56.53)
  line L262 (227.4425, -87.9625) -> (214.4425, -87.9625)
  line L263 (299.475, -41.125) -> (299.475, -54.125)
  line L264 (220.775, -66.055) -> (207.775, -66.055)
  line L265 (239.825, -23.48) -> (226.825, -23.48)
  line L266 (239.825, -37.48) -> (226.825, -37.48)
  line L267 (297.475, -41.125) -> (297.475, -54.125)
  arc A202 (214.4425, -73.9625) -> (213.9425, -74.4625) centre (214.4425, -74.4625) ccw
  line L268 (207.275, -52.555) -> (207.275, -65.555)
  arc A203 (227.9425, -74.4625) -> (227.4425, -73.9625) centre (227.4425, -74.4625) ccw
  line L269 (297.475, -41.125) -> (297.475, -54.125)
  line L270 (264.425, -39.22) -> (264.425, -52.22)
  line L271 (188.225, -54.46) -> (188.225, -67.46)
  line L272 (221.275, -52.555) -> (221.275, -65.555)
  line L273 (278.425, -39.22) -> (278.425, -52.22)
  line L274 (202.225, -54.46) -> (202.225, -67.46)
  arc A204 (220.775, -66.055) -> (221.275, -65.555) centre (220.775, -65.555) ccw
  line L275 (227.9425, -74.4625) -> (227.9425, -87.4625)
  line L276 (213.9425, -74.4625) -> (213.9425, -87.4625)
  line L277 (283.475, -41.125) -> (283.475, -54.125)
  line L278 (186.225, -54.46) -> (186.225, -65.0177)
  line L279 (245.375, -29.695) -> (245.375, -42.695)
  line L280 (204.2017, -76.0704) -> (207.5664, -88.6274)
  line L281 (201.725, -67.96) -> (188.725, -67.96)
  line L282 (259.375, -29.695) -> (259.375, -42.695)
  line L283 (203.5893, -75.7169) -> (191.0323, -79.0815)
  line L284 (207.275, -14.455) -> (207.275, -27.455)
  line L285 (186.225, -16.36) -> (186.225, -29.36)
  line L286 (277.925, -71.77) -> (264.925, -71.77)
  line L287 (176.8467, -103.5722) -> (189.1023, -96.4964)
  arc A205 (194.0434, -92.2509) -> (194.6558, -92.6045) centre (194.5264, -92.1215) ccw
  line L288 (167.6627, -85.6651) -> (174.1627, -96.9234)
  arc A206 (174.1627, -96.9234) -> (174.8457, -97.1064) centre (174.5957, -96.6734) ccw
  line L289 (174.8457, -97.1064) -> (186.104, -90.6064)
  line L290 (175.4806, -103.2062) -> (172.4306, -97.9234)
  arc A207 (167.8457, -84.9821) -> (167.6627, -85.6651) centre (168.0957, -85.4151) ccw
  line L291 (239.825, -18.43) -> (226.825, -18.43)
  arc A208 (179.787, -78.6651) -> (179.104, -78.4821) centre (179.354, -78.9151) ccw
  arc A209 (163.2467, -80.0163) -> (162.8806, -81.3823) centre (163.7467, -80.8823) ccw
  arc A210 (184.725, -67.6158) -> (186.225, -65.0177) centre (183.225, -65.0177) ccw
  arc A211 (188.225, -67.46) -> (188.725, -67.96) centre (188.725, -67.46) ccw
  arc A212 (191.0323, -79.0815) -> (190.6787, -79.6939) centre (191.1617, -79.5645) ccw
  line L292 (163.2467, -80.0163) -> (184.725, -67.6158)
  arc A213 (186.104, -90.6064) -> (186.287, -89.9234) centre (185.854, -90.1734) ccw
  arc A214 (175.4806, -103.2062) -> (176.8467, -103.5722) centre (176.3467, -102.7062) ccw
  arc A215 (190.1375, -96.1307) -> (189.1023, -96.4964) centre (190.6023, -99.0945) ccw
  point P0 (19.575, -19.575)
  point P1 (57.675, -8.145)
  point P2 (94.725, -13.86)
  point P3 (75.675, -11.955)
  point P4 (38.625, -17.67)
  point P5 (242.325, -8.145)
  point P6 (280.425, -19.575)
  point P7 (205.275, -13.86)
  point P8 (261.375, -17.67)
  point P9 (224.325, -11.955)
  point P10 (300, 0)
  dimension "d129" = 4
  dimension "d130" = 3
  dimension "d131" = 2
  dimension "d132" = 2
  dimension "d133" = 2
  dimension "d134" = 2
  dimension "d135" = 2
  dimension "d136" = 1
  dimension "d137" = 1
  dimension "d138" = 1
  dimension "d139" = 1
  dimension "d140" = 0.5
  dimension "d141" = 0.5
  dimension "d142" = 0.5
  dimension "d143" = 0.5
  dimension "d144" = 0.5
  dimension "d145" = 0.5
  dimension "d146" = 0.5
  dimension "d147" = 0.5
  dimension "d148" = 0.5
  dimension "d149" = 0.5
  dimension "d150" = 3
  dimension "d151" = 2
  dimension "d152" = 6.6
  dimension "d153" = 2
  dimension "d154" = 2
  dimension "d155" = 2
  dimension "d156" = 2
  dimension "d157" = 6.6
  dimension "d158" = 1
  dimension "d159" = 3
  dimension "d160" = 3
  dimension "d161" = 2
  dimension "d162" = 2
  dimension "d163" = 2
  dimension "d164" = 2
  dimension "d165" = 2
  dimension "d166" = 18
  dimension "d167" = 2
  constraint parallel L64 L89
  constraint parallel L70 L112
  constraint parallel L121 L123
  constraint parallel L39 L122
  constraint perpendicular L83 L89
  constraint parallel L31 L91
  constraint tangent L9 A78
  constraint tangent L64 A78
  constraint perpendicular L77 L87
  constraint perpendicular L76 L87
  constraint perpendicular L31 L86
  constraint perpendicular L36 L66
  constraint perpendicular L60 L66
  constraint perpendicular L93 L99
  constraint perpendicular L65 L93
  constraint perpendicular L22 L126
  constraint perpendicular L63 L68
  constraint perpendicular L90 L144
  constraint perpendicular L20 L90
  constraint perpendicular L61 L90
  constraint perpendicular L17 L61
  constraint perpendicular L21 L39
  constraint perpendicular L3 L108
  constraint tangent L76 A63
  constraint tangent L86 A63
  constraint tangent L73 A62
  constraint tangent A62 L89
  constraint tangent L14 A43
  constraint tangent A43 L70
  constraint tangent A14 L21
  constraint tangent L3 A14
  constraint tangent L66 A64
  constraint tangent L60 A64
  constraint coincident P0 L79
  constraint coincident P0 L66
  constraint tangent A48 L79
  constraint tangent L66 A48
  constraint coincident P4 L36
  constraint coincident P4 L93
  constraint tangent L36 A75
  constraint tangent A75 L93
  constraint tangent A67 L93
  constraint tangent L65 A67
  constraint coincident P1 L99
  constraint coincident P1 L22
  constraint tangent A32 L99
  constraint tangent L22 A32
  constraint tangent L22 A92
  constraint tangent L68 A92
  constraint tangent L90 A91
  constraint tangent L20 A91
  constraint coincident P3 L96
  constraint coincident P3 L90
  constraint tangent A57 L96
  constraint tangent A57 L90
  constraint tangent A31 L61
  constraint tangent L17 A31
  constraint coincident P2 L108
  constraint coincident P2 L17
  constraint tangent A19 L108
  constraint tangent A19 L17
  constraint tangent A17 L127
  constraint tangent A17 L14
  constraint parallel L36 L64
  constraint tangent A53 L98
  constraint tangent A53 L112
  constraint tangent A1 L9
  constraint tangent A1 L34
  constraint tangent L34 A86
  constraint tangent L98 A86
  constraint horizontal L43
  constraint vertical L10
  constraint horizontal L11
  constraint vertical L75
  constraint coincident L43.start L75.end
  constraint horizontal L106
  constraint vertical L71
  constraint horizontal L81
  constraint vertical L84
  constraint horizontal L57
  constraint vertical L114
  constraint horizontal L49
  constraint vertical L131
  constraint horizontal L132
  constraint vertical L117
  constraint horizontal L54
  constraint vertical L1
  constraint perpendicular L113 L143
  constraint coincident A35.centre L113.end
  constraint vertical L146
  constraint symmetric origin L146 P10
  constraint symmetric L36.start L146 L212.start
  constraint symmetric A55.start L146 A126.end
  constraint symmetric A70.end L146 A185.start
  constraint symmetric A1.start L146 A110.end
  constraint symmetric A1.end L146 A110.start
  constraint symmetric L9.end L146 L191.end
  constraint symmetric L64.end L146 L226.end
  constraint symmetric L86.end L146 L163.end
  constraint symmetric A32.start L146 L222.end
  constraint symmetric A67.end L146 L234.end
  constraint symmetric L65.start L146 L242.start
  constraint symmetric A76.end L146 A190.start
  constraint symmetric A20.start L146 A168.end
  constraint symmetric L67.start L146 A119.end
  constraint symmetric L134.start L146 L157.start
  constraint symmetric A34.end L146 A146.start
  constraint symmetric L35.end L146 A140.end
  constraint symmetric A6.end L146 L157.end
  constraint symmetric A6.start L146 A199.end
  constraint symmetric L48.end L146 A136.start
  constraint symmetric A34.start L146 L154.start
  constraint symmetric L142.end L146 L154.end
  constraint symmetric A84.end L146 A140.start
  constraint symmetric A13.start L146 L148.end
  constraint symmetric A40.end L146 L148.start
  constraint symmetric L70.end L146 L150.end
  constraint symmetric A15.end L146 L192.start
  constraint symmetric A23.start L146 L192.end
  constraint symmetric L69.start L146 A119.start
  constraint symmetric A15.start L146 L217.end
  constraint symmetric A35.centre L146 L200.end
  constraint symmetric L20.start L146 L170.start
  constraint symmetric A31.end L146 A116.start
  constraint symmetric L17.start L146 L156.start
  constraint symmetric A57.end L146 L172.start
  constraint symmetric L90.end L146 L158.end
  constraint symmetric A57.start L146 L158.start
  constraint symmetric L98.end L146 L287.end
  constraint symmetric L34.end L146 L213.end
  constraint symmetric L86.start L146 L163.start
  constraint symmetric L76.end L146 A142.start
  constraint symmetric L73.end L146 L168.end
  constraint symmetric L25.end L146 L179.end
  constraint symmetric A54.end L146 A188.start
  constraint symmetric A28.end L146 A176.start
  constraint symmetric A33.start L146 A134.end
  constraint symmetric L48.start L146 A188.end
  constraint symmetric A33.end L146 L179.start
  constraint symmetric A28.start L146 A176.end
  constraint symmetric A19.start L146 L156.end
  constraint symmetric A17.end L146 A210.start
  constraint symmetric A17.start L146 L278.end
  constraint symmetric A19.end L146 A118.start
  constraint symmetric L8.end L146 A111.end
  constraint symmetric A25.end L146 A111.start
  constraint symmetric A4.end L146 A193.start
  constraint symmetric A65.start L146 L272.end
  constraint symmetric A3.start L146 A197.end
  constraint symmetric A62.end L146 L166.start
  constraint symmetric A43.start L146 L150.start
  constraint symmetric L113.start L146 L200.start
  constraint symmetric L14.start L146 A209.start
  constraint symmetric A30.end L146 A149.start
  constraint symmetric L8.start L146 L264.start
  constraint symmetric A3.end L146 L176.end
  constraint symmetric A23.end L146 A172.start
  constraint symmetric A30.start L146 A149.end
  constraint symmetric A4.start L146 L176.start
  constraint symmetric L118.start L146 L169.start
  constraint symmetric L38.start L146 A201.start
  constraint symmetric L38.end L146 L281.end
  constraint symmetric A44.end L146 L271.end
  constraint symmetric A0.start L146 A121.end
  constraint symmetric A0.end L146 A121.start
  constraint symmetric L40.start L146 A173.start
  constraint symmetric L40.end L146 A201.end
  constraint symmetric A60.start L146 L201.end
  constraint symmetric L12.start L146 A138.end
  constraint symmetric A80.end L146 A138.start
  constraint symmetric L12.end L146 L218.end
  constraint symmetric L46.start L146 L228.start
  constraint symmetric L46.end L146 L228.end
  constraint symmetric L60.start L146 A141.end
  constraint symmetric L66.end L146 A141.start
  constraint symmetric L3.start L146 L167.start
  constraint symmetric A14.end L146 L162.end
  constraint symmetric A48.start L146 L188.end
  constraint symmetric L66.start L146 L187.start
  constraint symmetric A53.start L146 L287.start
  constraint symmetric A53.end L146 L290.start
  constraint symmetric A56.end L146 L178.end
  constraint symmetric A7.end L146 L189.start
  constraint symmetric L19.start L146 L190.start
  constraint symmetric L19.end L146 L190.end
  constraint symmetric A61.start L146 L178.start
  constraint symmetric L82.end L146 A139.end
  constraint symmetric A7.start L146 A150.end
  constraint symmetric L74.start L146 A170.start
  constraint symmetric A56.start L146 L165.start
  constraint symmetric L80.end L146 L165.end
  constraint symmetric A75.end L146 L234.start
  constraint symmetric L36.end L146 L212.end
  constraint symmetric L16.start L146 L229.start
  constraint symmetric L16.end L146 L229.end
  constraint symmetric L4.start L146 A166.start
  constraint symmetric L4.end L146 A167.end
  constraint symmetric L5.start L146 A169.end
  constraint symmetric L5.end L146 A167.start
  constraint symmetric A12.start L146 A166.end
  constraint symmetric L15.start L146 L240.start
  constraint symmetric A27.end L146 A112.start
  constraint symmetric A69.end L146 A200.start
  constraint symmetric A27.start L146 A112.end
  constraint symmetric L95.start L146 L259.start
  constraint symmetric A69.start L146 L259.end
  constraint symmetric L27.start L146 L260.start
  constraint symmetric L29.start L146 A202.end
  constraint symmetric L27.end L146 L260.end
  constraint symmetric L2.start L146 L160.start
  constraint symmetric L125.end L146 L254.end
  constraint symmetric L125.start L146 L254.start
  constraint symmetric A101.end L146 A194.start
  constraint symmetric A104.start L146 L180.start
  constraint symmetric A5.start L146 L160.end
  constraint symmetric L140.end L146 A196.end
  constraint symmetric A5.end L146 A127.start
  constraint symmetric L28.start L146 A179.start
  constraint symmetric L28.end L146 A145.end
  constraint symmetric A49.end L146 L196.end
  constraint symmetric A29.start L146 L196.start
  constraint symmetric A29.end L146 L185.start
  constraint symmetric A49.start L146 L198.start
  constraint symmetric A66.end L146 A145.start
  constraint symmetric L77.end L146 L185.end
  constraint symmetric A16.end L146 L283.end
  constraint symmetric A22.end L146 A109.start
  constraint symmetric L37.end L146 L220.end
  constraint symmetric L41.start L146 A108.start
  constraint symmetric A22.start L146 A109.end
  constraint symmetric L58.start L146 A108.end
  constraint symmetric A37.end L146 L152.end
  constraint symmetric A10.start L146 A133.end
  constraint symmetric A26.start L146 L152.start
  constraint symmetric A73.end L146 A165.start
  constraint symmetric L7.start L146 A162.start
  constraint symmetric L7.end L146 A154.end
  constraint symmetric A93.end L146 A124.start
  constraint symmetric A71.end L146 A154.start
  constraint symmetric A24.start L146 A162.end
  constraint symmetric A105.start L146 A195.end
  constraint symmetric L18.start L146 L171.start
  constraint symmetric A10.end L146 L171.end
  constraint symmetric A47.start L146 L209.start
  constraint symmetric A26.end L146 A155.start
  constraint symmetric L92.end L146 A165.end
  constraint symmetric A52.end L146 L288.end
  constraint symmetric A81.end L146 L149.end
  constraint symmetric A13.end L146 L147.start
  constraint symmetric A40.start L146 L288.start
  constraint symmetric A16.start L146 L149.start
  constraint symmetric L44.start L146 A124.end
  constraint symmetric A38.end L146 L215.end
  constraint symmetric A18.start L146 L215.start
  constraint symmetric L44.end L146 L241.end
  constraint symmetric A11.end L146 A174.start
  constraint symmetric L26.start L146 A206.end
  constraint symmetric L24.end L146 L147.end
  constraint symmetric P0 L146 P6
  constraint symmetric L79.start L146 L188.start
  constraint symmetric L26.end L146 L289.end
  constraint symmetric A36.start L146 A153.end
  constraint symmetric A8.end L146 L223.end
  constraint symmetric A36.end L146 L209.end
  constraint symmetric A21.end L146 A152.start
  constraint symmetric L6.start L146 L211.start
  constraint symmetric L6.end L146 L211.end
  constraint symmetric A8.start L146 L219.end
  constraint symmetric L33.end L146 A160.start
  constraint symmetric A18.end L146 A159.start
  constraint symmetric A11.start L146 A174.end
  constraint symmetric A38.start L146 A158.end
  constraint symmetric L13.end L146 A160.end
  constraint symmetric L73.start L146 L168.start
  constraint symmetric L47.start L146 L194.start
  constraint symmetric L68.end L146 L153.start
  constraint symmetric L39.end L146 L182.end
  constraint symmetric L3.end L146 L167.end
  constraint symmetric P1 L146 P5
  constraint symmetric P2 L146 P7
  constraint symmetric L20.end L146 L153.end
  constraint symmetric L21.start L146 L162.start
  constraint symmetric L31.end L146 L183.end
  constraint symmetric L121.end L146 L199.end
  constraint symmetric L121.start L146 L199.start
  constraint symmetric L122.start L146 L182.start
  constraint symmetric L31.start L146 L183.start
  constraint symmetric L65.end L146 L222.start
  constraint symmetric L47.end L146 L247.end
  constraint symmetric L64.start L146 L166.end
  constraint symmetric L102.end L146 L177.end
  constraint symmetric L124.start L146 A137.start
  constraint symmetric L56.end L146 A137.end
  constraint symmetric A41.start L146 L177.start
  constraint symmetric L124.end L146 A117.end
  constraint symmetric A41.end L146 A132.start
  constraint symmetric L42.start L146 A131.end
  constraint symmetric L119.start L146 A120.start
  constraint symmetric L120.end L146 L173.end
  constraint symmetric A94.start L146 L206.end
  constraint symmetric L0.start L146 A147.start
  constraint symmetric L0.end L146 A120.end
  constraint symmetric L115.start L146 L161.start
  constraint symmetric A94.end L146 L161.end
  constraint symmetric A2.start L146 L173.start
  constraint symmetric A9.start L146 A115.end
  constraint symmetric L51.end L146 A123.end
  constraint symmetric L53.end L146 A189.start
  constraint symmetric A95.end L146 A123.start
  constraint symmetric L51.start L146 A114.start
  constraint symmetric A83.start L146 A114.end
  constraint symmetric A9.end L146 A115.start
  constraint symmetric A96.start L146 A189.end
  constraint symmetric L42.end L146 A117.start
  constraint symmetric L55.end L146 L210.end
  constraint symmetric A20.end L146 A168.start
  constraint symmetric L55.start L146 A126.start
  constraint symmetric L30.start L146 L238.start
  constraint symmetric P3 L146 P9
  constraint symmetric P4 L146 P8
  constraint symmetric L61.start L146 L172.end
  constraint symmetric L49.end L146 L181.end
  constraint symmetric L57.start L146 A117.centre
  constraint symmetric L49.start L146 L155.end
  constraint symmetric L57.end L146 L155.start
  constraint symmetric L68.start L146 L221.start
  constraint symmetric L22.start L146 L233.start
  constraint symmetric L22.end L146 A163.start
  constraint symmetric L71.start L146 L175.end
  constraint symmetric A56.centre L146 L184.end
  constraint symmetric L10.start L146 L214.end
  constraint symmetric L11.end L146 L197.start
  constraint symmetric L43.start L146 A145.centre
  constraint symmetric L10.end L146 L225.start
  constraint symmetric L84.end L146 L175.start
  constraint symmetric L71.end L146 L184.start
  constraint symmetric L54.start L146 L174.end
  constraint symmetric L117.start L146 L174.start
  constraint symmetric A5.centre L146 A127.centre
  constraint symmetric A3.centre L146 L186.end
  constraint symmetric A0 L146 A121
  constraint symmetric A1 L146 A110
  constraint symmetric A2 L146 A147
  constraint symmetric A3 L146 A197
  constraint symmetric A4 L146 A193
  constraint symmetric A5 L146 A127
  constraint symmetric A6 L146 A199
  constraint symmetric A7 L146 A150
  constraint symmetric A8 L146 A157
  constraint symmetric A9 L146 A115
  constraint symmetric A10 L146 A133
  constraint symmetric A11 L146 A174
  constraint symmetric A12 L146 A166
  constraint symmetric A13 L146 A208
  constraint symmetric A14 L146 A122
  constraint symmetric A15 L146 A156
  constraint symmetric A16 L146 A212
  constraint symmetric A17 L146 A210
  constraint symmetric A18 L146 A159
  constraint symmetric A19 L146 A118
  constraint symmetric A20 L146 A168
  constraint symmetric A21 L146 A152
  constraint symmetric A22 L146 A109
  constraint symmetric A23 L146 A172
  constraint symmetric A24 L146 A162
  constraint symmetric A25 L146 A111
  constraint symmetric A26 L146 A155
  constraint symmetric A27 L146 A112
  constraint symmetric A28 L146 A176
  constraint symmetric A29 L146 A180
  constraint symmetric A30 L146 A149
  constraint symmetric A31 L146 A116
  constraint symmetric A32 L146 A182
  constraint symmetric A33 L146 A134
  constraint symmetric A34 L146 A146
  constraint symmetric A35 L146 A178
  constraint symmetric A36 L146 A153
  constraint symmetric A37 L146 A128
  constraint symmetric A38 L146 A158
  constraint symmetric A39 L146 A167
  constraint symmetric A40 L146 A207
  constraint symmetric A41 L146 A132
  constraint symmetric A42 L146 A113
  constraint symmetric A43 L146 A209
  constraint symmetric A44 L146 A211
  constraint symmetric A45 L146 A201
  constraint symmetric A46 L146 A187
  constraint symmetric A47 L146 A171
  constraint symmetric A48 L146 A148